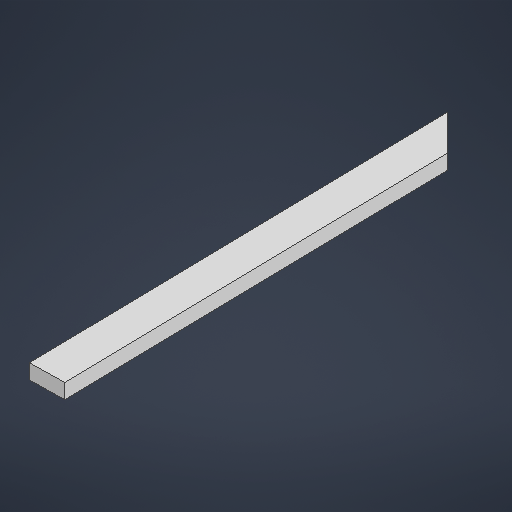
# Autodesk Inventor part: S_2x4x42.997
Saved by Autodesk Inventor 2026 (Build 300175000, 175)
## iProperties
Created: 2025-09-08
Part Number: S_2x4x42.997
Material: Generic
Document SubType Name: Modeling
Designer: trott
Density: 1 g/cm^3
Appearance: Default
Author: trott
Autodesk Inventor part; units mm, degrees
ref_plane "YZ Plane" through (0, 0, 0) normal (1, 0, 0) x (0, 1, 0)
ref_plane "XZ Plane" through (0, 0, 0) normal (0, 1, 0) x (-1, 0, 0)
ref_plane "XY Plane" through (0, 0, 0) normal (0, 0, 1) x (1, 0, 0)
sketch "Sketch1" plane through (0, 0, 0) normal (0, 1, 0) x (-1, 0, 0)
  line L0 (0, 0) -> (0, -1219.2)
  line L1 (0, 0) -> (88.9, 0)
  line L2 (88.9, 0) -> (88.9, -1219.2)
  line L3 (88.9, -1219.2) -> (0, -1219.2)
  line L4 (0, 0) -> (0, 1219.2) construction
  line L5 (0, 1219.2) -> (1219.2, 1219.2) construction
  line L6 (0, 1219.2) -> (0, 3657.6) construction
  line L7 (0, 3657.6) -> (0, 4876.8) construction
  line L8 (0, 4876.8) -> (0, 6096) construction
  line L9 (0, -1219.2) -> (2438.4, -1219.2) construction
  line L10 (0, 6096) -> (2438.4, 6096) construction
  line L11 (2438.4, 6096) -> (2438.4, -1219.2) construction
  line L12 (0, 3657.6) -> (0, 3352.8) construction
  line L13 (0, 3352.8) -> (2438.4, 3352.8) construction
  line L14 (2438.4, 3352.8) -> (1219.2, 3352.8)
  line L15 (1219.2, 3352.8) -> (1219.2, 3263.9)
  line L16 (1219.2, 3263.9) -> (2438.4, 3263.9)
  line L17 (2438.4, 3263.9) -> (2438.4, 3352.8)
  line L18 (0, 6096) -> (862.1046, 6958.1046)
  line L19 (862.1046, 6958.1046) -> (924.9664, 6895.2428)
  line L20 (924.9664, 6895.2428) -> (62.8618, 6033.1382)
  line L21 (62.8618, 6033.1382) -> (0, 6096)
  line L22 (0, 4876.8) -> (1219.2, 4876.8) construction
  line L23 (1219.2, 4876.8) -> (2081.3046, 5738.9046)
  line L24 (1219.2, 1219.2) -> (2081.3046, 357.0954)
  line L25 (2081.3046, 357.0954) -> (2018.4428, 294.2336)
  line L26 (2018.4428, 294.2336) -> (1156.3382, 1156.3382)
  line L27 (1156.3382, 1156.3382) -> (1219.2, 1219.2)
  line L28 (2018.4428, 294.2336) -> (88.9, -1219.2)
  line L29 (2081.3046, 357.0954) -> (2144.1664, 419.9572)
  line L30 (2144.1664, 419.9572) -> (1282.0618, 1282.0618)
  line L31 (1282.0618, 1282.0618) -> (1219.2, 1219.2)
  line L32 (2438.4, 3352.8) -> (2438.4, 3441.7)
  line L33 (2438.4, 3441.7) -> (1219.2, 3441.7)
  line L34 (1219.2, 3441.7) -> (1219.2, 3352.8)
  line L35 (1156.3382, 4939.6618) -> (1282.0618, 4813.9382)
  line L36 (2018.4428, 5801.7664) -> (2144.1664, 5676.0428)
  line L37 (1282.0618, 4813.9382) -> (2144.1664, 5676.0428)
  line L38 (2018.4428, 5801.7664) -> (1156.3382, 4939.6618)
  line L39 (2018.4428, 5801.7664) -> (924.9664, 6895.2428)
  line L40 (62.8618, 6033.1382) -> (1156.3382, 4939.6618)
  line L41 (1233.6206, 4168.8855) -> (1267.6412, 4086.7527)
  line L42 (1263.7078, 2313.9849) -> (1230.0006, 2231.7229)
  arc A0 (862.1046, 6958.1046) -> (0, 6096) centre (431.0523, 6527.0523) ccw
  line L43 (1246.8542, 2272.8539) -> (2375.0183, 1810.583)
  line L44 (2391.8719, 1851.7139) -> (2358.1646, 1769.452)
  line L45 (2391.8719, 1851.7139) -> (1263.7078, 2313.9849)
  line L46 (1230.0006, 2231.7229) -> (2358.1646, 1769.452)
  line L47 (1230.0006, 2231.7229) -> (1219.2, 3263.9)
  line L48 (2144.1664, 419.9572) -> (2391.8719, 1851.7139)
  line L49 (2391.8719, 1851.7139) -> (2438.4, 3263.9)
  line L50 (1219.2, 3441.7) -> (1233.6206, 4168.8855)
  line L51 (1250.6309, 4127.8191) -> (2377.0248, 4594.3867)
  line L52 (2360.0145, 4635.4532) -> (2394.0351, 4553.3203)
  line L53 (2394.0351, 4553.3203) -> (1267.6412, 4086.7527)
  line L54 (2360.0145, 4635.4532) -> (1233.6206, 4168.8855)
  line L55 (2394.0351, 4553.3203) -> (2144.1664, 5676.0428)
  line L56 (2438.4, 3441.7) -> (2394.0351, 4553.3203)
  line L57 (2144.1664, 5676.0428) -> (2057.3895, 5656.7301)
  line L58 (2394.0351, 4553.3203) -> (2305.2058, 4549.7751)
  line L59 (2394.0351, 4553.3203) -> (2307.2582, 4534.0076)
  line L60 (2307.2582, 4534.0076) -> (2057.3895, 5656.7301)
  line L61 (2438.4, 3441.7) -> (2349.5707, 3438.1548)
  line L62 (2349.5707, 3438.1548) -> (2305.2058, 4549.7751)
  line L63 (1219.2, 3441.7) -> (1308.0825, 3439.9374)
  line L64 (1233.6206, 4168.8855) -> (1322.5031, 4167.1229)
  line L65 (1322.5031, 4167.1229) -> (1308.0825, 3439.9374)
  line L66 (2018.4428, 5801.7664) -> (1955.581, 5738.9046)
  line L67 (1955.581, 5738.9046) -> (862.1046, 6832.381)
  line L68 (924.9664, 6895.2428) -> (862.1046, 6832.381)
  line L69 (62.8618, 6033.1382) -> (125.7236, 6096)
  line L70 (62.8618, 6033.1382) -> (125.7236, 6096)
  line L71 (125.7236, 6096) -> (1219.2, 5002.5236)
  line L72 (1156.3382, 1156.3382) -> (0, 0)
  line L73 (0, 0) -> (62.8618, -62.8618)
  line L74 (1156.3382, 1156.3382) -> (1219.2, 1093.4764)
  line L75 (1219.2, 1093.4764) -> (62.8618, -62.8618)
  line L76 (2018.4428, 294.2336) -> (1963.5776, 364.1837)
  line L77 (88.9, -1219.2) -> (34.0348, -1149.2499)
  line L78 (34.0348, -1149.2499) -> (1963.5776, 364.1837)
  line L79 (2144.1664, 419.9572) -> (2056.5677, 435.1125)
  line L80 (2391.8719, 1851.7139) -> (2304.2732, 1866.8692)
  line L81 (2391.8719, 1851.7139) -> (2303.0201, 1854.6414)
  line L82 (2304.2732, 1866.8692) -> (2056.5677, 435.1125)
  line L83 (1230.0006, 2231.7229) -> (1318.8957, 2232.6531)
  line L84 (1219.2, 3263.9) -> (1308.0951, 3264.8302)
  line L85 (1308.0951, 3264.8302) -> (1318.8957, 2232.6531)
  line L86 (2438.4, 3263.9) -> (2349.5482, 3266.8275)
  line L87 (2349.5482, 3266.8275) -> (2303.0201, 1854.6414)
  line L88 (88.9, 0) -> (125.7236, 0)
  line L89 (1233.6206, 4168.8855) -> (1219.2, 4876.8)
  line L90 (1233.6206, 4168.8855) -> (1322.5022, 4170.6961)
  line L91 (1219.2, 4876.8) -> (1308.0816, 4878.6106)
  line L92 (1308.0816, 4878.6106) -> (1322.5022, 4170.6961)
  line L93 (1282.0618, 4813.9382) -> (1309.9674, 4786.0326)
  line L94 (1267.6412, 4086.7527) -> (1318.4756, 3964.0275)
  line L95 (2360.0145, 4635.4532) -> (2374.4273, 4641.4231)
  line L96 (1230.0006, 2231.7229) -> (1219.2, 1219.2)
  line L97 (1230.0006, 2231.7229) -> (1318.8955, 2230.7747)
  line L98 (1219.2, 1219.2) -> (1308.0949, 1218.2518)
  line L99 (1308.0949, 1218.2518) -> (1318.8955, 2230.7747)
  line L100 (1282.0618, 1282.0618) -> (1309.0636, 1309.0636)
  line L101 (1263.7078, 2313.9849) -> (1316.7428, 2438.4)
  line L102 (2358.1646, 1769.452) -> (2376.5379, 1763.082)
  line L103 (2286, 3352.8) -> (1371.6, 3352.8)
  line L104 (2286, 3441.7) -> (2286, 3263.9)
  line L105 (1371.6, 3441.7) -> (1371.6, 3263.9)
  line L106 (0, -152.4) -> (0, -1066.8)
  line L107 (0, -152.4) -> (88.9, -152.4)
  line L108 (0, -1066.8) -> (88.9, -1066.8)
  line L109 (1326.9631, 1111.4369) -> (1973.5415, 464.8585)
  line L110 (2036.4033, 527.7203) -> (1910.6797, 401.9967)
  line L111 (1389.8249, 1174.2987) -> (1264.1013, 1048.5751)
  line L112 (2233.9978, 1868.3668) -> (1387.8747, 2215.07)
  line L113 (1404.7283, 2256.201) -> (1371.0211, 2173.939)
  line L114 (2250.8514, 1909.4978) -> (2217.1441, 1827.2358)
  line L115 (1371.0211, 2173.939) -> (1389.8249, 1174.2987)
  line L116 (1264.1013, 1048.5751) -> (88.9, -152.4)
  line L117 (2217.1441, 1827.2358) -> (2036.4033, 527.7203)
  line L118 (1910.6797, 401.9967) -> (88.9, -1066.8)
  line L119 (88.9, -1066.8) -> (33.1016, -997.592)
  line L120 (1910.6797, 401.9967) -> (1854.8813, 471.2047)
  line L121 (1854.8813, 471.2047) -> (33.1016, -997.592)
  line L122 (88.9, -152.4) -> (0, -243.2497)
  line L123 (0, -243.2497) -> (63.5399, -305.426)
  line L124 (1263.7078, 1048.9686) -> (1327.2477, 986.7923)
  line L125 (1327.2477, 986.7923) -> (88.9, -278.7141)
  line L126 (1389.8249, 1174.2987) -> (1392.2351, 1046.1649)
  line L127 (1392.2351, 1046.1649) -> (1481.1194, 1047.8368)
  line L128 (1371.0211, 2173.939) -> (1459.9053, 2175.611)
  line L129 (1459.9053, 2175.611) -> (1460.6275, 2137.2224)
  line L130 (2036.4033, 527.7203) -> (1948.3509, 539.9669)
  line L131 (2217.1441, 1827.2358) -> (2223.465, 1872.6827)
  line L132 (2223.465, 1872.6827) -> (2135.4126, 1884.9293)
  line L133 (2135.4126, 1884.9293) -> (2132.2278, 1862.0307)
  line L134 (88.9, -278.7141) -> (63.1422, -305.0368)
  line L135 (2132.2278, 1862.0307) -> (1948.3509, 539.9669)
  line L136 (1480.4452, 1083.6784) -> (1481.1194, 1047.8368)
  line L137 (1460.6275, 2137.2224) -> (1480.4452, 1083.6784)
  point P0 (1955.1236, 357.5528)
  point P1 (88.9, -1106.2164)
  point P2 (2292.1025, 1796.5213)
  point P3 (2067.2525, 496.8711)
  point P4 (1318.5187, 2195.4522)
  point P5 (1308.1049, 3263.9)
  point P6 (2349.4518, 3263.9)
  point P7 (2304.1085, 1887.6754)
  point P8 (2306.5112, 4517.0667)
  point P9 (2349.4292, 3441.7)
  point P10 (1308.1175, 3441.7)
  point P11 (2069.6708, 5601.5472)
  point P12 (2291.0394, 4606.8827)
  point P13 (1321.7951, 4205.4086)
  point P14 (1828.8, 3352.8)
  point P15 (0, -609.6)
  point P16 (1650.2523, 788.1477)
  point P17 (1810.9362, 2041.7184)
  point P18 (88.9, -278.7141)
  point P19 (1326.5733, 986.1031)
  point P20 (1957.6068, 606.5167)
  point P21 (1957.6068, 606.5167)
  point P22 (1480.4452, 1083.6784)
  dimension "d0" = 1219.2
  dimension "d2" = 1219.2
  dimension "d3" = 1219.2
  dimension "d16" = 2438.4
  dimension "d17" = 1219.2
  dimension "d18" = 1219.2
  dimension "d20" = 2438.4
  dimension "d21" = 304.8
  dimension "d22" = 1219.2
  dimension "d23" = 88.9
  dimension "d24" = 1219.2
  dimension "d25" = 45
  dimension "d26" = 88.9
  dimension "d27" = 1219.2
  dimension "d28" = 1219.2
  dimension "d29" = 1219.2
  dimension "d31" = 1219.2
  dimension "d32" = 88.9
  dimension "d33" = 88.9
  dimension "d34" = 88.9
  dimension "d35" = 177.8
  dimension "d36" = 177.8
  dimension "d38" = 88.9
  dimension "d39" = 88.9
  dimension "d43" = 1219.2
  dimension "d44" = 88.9
  dimension "d45" = 1219.2
  dimension "d46" = 88.9
  dimension "d47" = 88.9
  dimension "d48" = 88.9
  dimension "d49" = 88.9
  dimension "d50" = 88.9
  dimension "d51" = 88.9
  dimension "d54" = 88.9
  dimension "d55" = 88.9
  dimension "d57" = 88.9
  dimension "d58" = 88.9
  dimension "d59" = 88.9
  dimension "d60" = 88.9
  dimension "d61" = 88.9
  dimension "d64" = 88.9
  dimension "d65" = 88.9
  dimension "d66" = 88.9
  dimension "d69" = 88.9
  dimension "d70" = 88.9
  dimension "d71" = 88.9
  dimension "d72" = 88.9
  dimension "d73" = 914.4
  dimension "d74" = 914.4
  dimension "d75" = 914.4
  dimension "d76" = 914.4
  dimension "d77" = 88.9
  dimension "d78" = 88.9
  dimension "d79" = 88.9
  dimension "d80" = 88.9
  dimension "d83" = 88.9
  dimension "d84" = 88.9
  dimension "d85" = 88.9
  dimension "d86" = 88.9
  constraints: 276 end point, 61 perpendicular, 40 point on line, 22 midpoint, 6 horizontal, 3 collinear, 3 parallel, 2 point on circle, 2 vertical, 1 centre point
  measures "d0" distance of L0.start L0.end
  measures "d2" distance of L0.start L4.end
  measures "d3" distance of L4.end L5.end
  measures "d16" distance of L4.end L6.end
  measures "d17" distance of L6.end L7.end
  measures "d18" distance of L8.end L7.end
  measures "d20" distance of L8.end L10.end
  measures "d21" distance of L6.end L12.end
  measures "d22" distance of L13.end L14.end
  measures "d23" distance of L14.end L15.end
  measures "d24" distance of L8.end L18.end
  measures "d25" angle of L10 L18
  measures "d26" distance of L18.end L19.end
  measures "d27" distance of L19.end L20.end
  measures "d28" distance of L7.end L22.end
  measures "d29" distance of L22.end L23.end
  measures "d31" distance of L5.end L24.end
  measures "d32" distance of L24.end L25.end
  measures "d33" distance of L24.end L29.end
  measures "d34" distance of L13.end L32.end
  measures "d35" distance of L35.start L35.end
  measures "d36" distance of L36.start L36.end
  measures "d38" distance of L41.start L41.end
  measures "d39" distance of L42.start L42.end
  measures "d43" distance of L43.start L43.end
  measures "d44" distance of L44.start L44.end
  measures "d45" distance of L51.start L51.end
  measures "d46" distance of L36.end L57.end
  measures "d47" distance of L52.end L58.end
  measures "d48" distance of L52.end L59.end
  measures "d49" distance of L32.end L61.end
  measures "d50" distance of L33.end L63.end
  measures "d51" distance of L41.start L64.end
  measures "d54" distance of L20.end L69.end
  measures "d55" distance of L26.end L74.end
  measures "d57" distance of L25.end L76.end
  measures "d58" distance of L2.end L77.end
  measures "d59" distance of L29.end L79.end
  measures "d60" distance of L44.start L80.end
  measures "d61" distance of L44.start L81.end
  measures "d64" distance of L42.end L83.end
  measures "d65" distance of L15.end L84.end
  measures "d66" distance of L16.end L86.end
  measures "d69" distance of L41.start L90.end
  measures "d70" distance of L22.end L91.end
  measures "d71" distance of L42.end L97.end
  measures "d72" distance of L5.end L98.end
  measures "d73" distance of L103.start L103.end
  measures "d74" distance of L106.start L106.end
  measures "d75" distance of L109.start L109.end
  measures "d76" distance of L112.start L112.end
  measures "d77" distance of L108.end L119.end
  measures "d78" distance of L110.end L120.end
  measures "d79" distance of L122.end L123.end
  measures "d80" distance of L124.start L124.end
  measures "d83" distance of L126.end L127.end
  measures "d84" distance of L113.end L128.end
  measures "d85" distance of L110.start L130.end
  measures "d86" distance of L131.end L132.end
extrude "Extrusion2" add sketch "Sketch1" along normal blind 38.1 contours L115 L46 L137 L30 | L128 L129 L46
body "Solid2"
